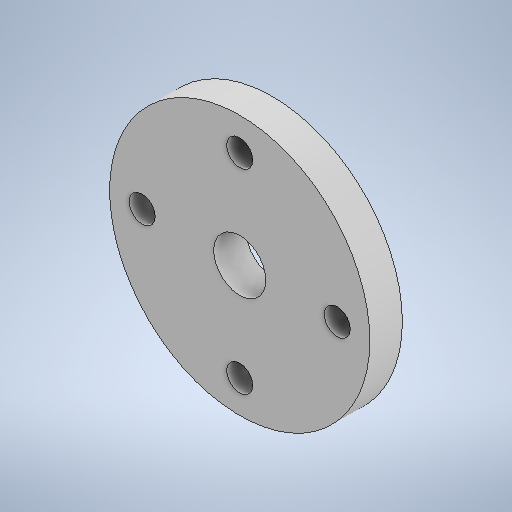
# Autodesk Inventor part: Brida1
Saved by Autodesk Inventor 2026 (Build 300175050, 175E)
## iProperties
Created: 2025-07-05
Part Number: Brida1
Material: Genérico
Document SubType Name: Modeling
Designer: piero
Density: 1 g/cm^3
Appearance: Valor por defecto
Author: piero
Autodesk Inventor part; units mm, degrees
ref_plane "YZ Plane" through (0, 0, 0) normal (1, 0, 0) x (0, 1, 0)
ref_plane "XZ Plane" through (0, 0, 0) normal (0, 1, 0) x (-1, 0, 0)
ref_plane "XY Plane" through (0, 0, 0) normal (0, 0, 1) x (1, 0, 0)
sketch "Boceto1" plane through (0, 0, 0) normal (0, 0, 1) x (1, 0, 0)
  circle A0 centre (0, 0) radius 20
  circle A1 centre (0, 0) radius 4
  dimension "d0" = 40
  dimension "d42" = 8
  constraints: 2 centre point, 2 coincident
  measures "d0" diameter of A0
  measures "d42" diameter of A1
extrude "Extrusión1" add sketch "Boceto1" along normal blind 5
sketch "Boceto3" plane through (0, 0, 0) normal (0, 0, -1) x (-1, 0, 0)
  circle A0 centre (0, 15) radius 2
  circle A1 centre (-15, 0) radius 2
  circle A2 centre (15, 0) radius 2
  circle A3 centre (0, -15) radius 2
  point P0 (0, 0)
  dimension "d6" = 4
  dimension "d7" = 4
  dimension "d8" = 4
  dimension "d9" = 4
  dimension "d10" = 15
  dimension "d11" = 15
  dimension "d12" = 15
  dimension "d13" = 15
  constraints: 4 centre point
  measures "d6" diameter of A0
  measures "d7" diameter of A1
  measures "d8" diameter of A2
  measures "d9" diameter of A3
  measures "d10" distance of A0.centre point (0, 0)
  measures "d11" distance of A3.centre point (0, 0)
  measures "d12" distance of point (0, 0) A1.centre
  measures "d13" distance of A2.centre point (0, 0)
hole "Agujero1" at (0, 15, 0) direction (0, 0, 1) diameter 4 end through all
hole "Agujero2" at (15, 0, 0) direction (0, 0, 1) diameter 4 end through all
hole "Agujero3" at (-15, 0, 0) direction (0, 0, 1) diameter 4 end through all
hole "Agujero4" at (0, -15, 0) direction (0, 0, 1) diameter 4 end through all
